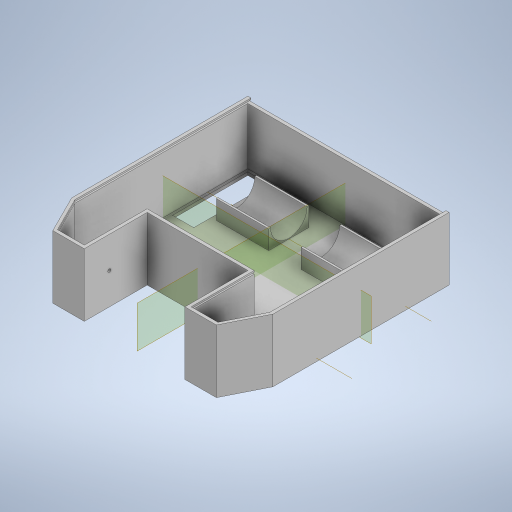
# Autodesk Inventor part: Bot v1 bottom
Saved by Autodesk Inventor 2024 (Build 280153000, 153)
## iProperties
Created: 2023-09-24
Part Number: Bot v1 bottom
Material: PBT Plastic
Document SubType Name: Modeling
Designer: CJ110
Density: 1.31 g/cm^3
Appearance: Smooth - White
Mass: 388.228 g
Surface Area: 1967.58 cm^2
Volume: 296.357 cm^3
Author: CJ110
Autodesk Inventor part; units mm, degrees
ref_plane "YZ Plane" through (0, 0, 0) normal (1, 0, 0) x (0, 1, 0)
sketch "Sketch1" plane through (0, 0, 0) normal (0, 1, 0) x (-1, 0, 0)
  line L0 (0, 0) -> (177.8, 0)
  line L1 (177.8, 0) -> (177.8, 203.2)
  line L2 (177.8, 203.2) -> (0, 203.2)
  line L3 (0, 203.2) -> (0, 0)
  dimension "Body_Length" = 177.8
  dimension "Body_Width" = 203.2
  constraints: 8 end point, 2 parallel, 1 horizontal, 1 perpendicular
  measures "Body_Length" distance of L0.start L0.end
  measures "Body_Width" distance of L2.end L0.start
extrude "Base" add sketch "Sketch1" along normal blind 3.175
sketch "Sketch3" plane through (0, 0, 0) normal (0, 1, 0) x (1, 0, 0)
  line L0 (-177.8, 0) -> (-177.8, -203.2) projected
  line L1 (-177.8, -203.2) -> (0, -203.2) projected
  line L2 (0, -203.2) -> (0, 0) projected
  line L3 (0, 0) -> (-177.8, 0) projected
  line L4 (-174.625, -3.175) -> (-3.175, -3.175)
  line L5 (-3.175, -3.175) -> (-3.175, -200.025)
  line L6 (-3.175, -200.025) -> (-174.625, -200.025)
  line L7 (-174.625, -200.025) -> (-174.625, -155.575)
  line L8 (-152.4, -152.4) -> (-152.4, -50.8)
  line L9 (-174.625, -47.625) -> (-174.625, -3.175)
  line L10 (-177.8, 0) -> (-177.8, -203.2) projected
  line L11 (-174.625, -155.575) -> (-149.225, -155.575)
  line L12 (-149.225, -155.575) -> (-149.225, -47.625)
  line L13 (-149.225, -47.625) -> (-174.625, -47.625)
  line L14 (-152.4, -152.4) -> (-177.8, -152.4)
  line L15 (-152.4, -50.8) -> (-177.8, -50.8)
  dimension "Wall_Thickness" = 3.175
  dimension "Cuttout_Width" = 101.6
  dimension "Cuttout_Depth" = 25.4
  dimension "d30" = 3.175
  dimension "d31" = 3.175
  dimension "d32" = 3.175
  dimension "d33" = 3.175
  constraints: 22 end point, 5 perpendicular, 3 point on line, 2 vertical, 1 collinear, 2 other
  measures "Wall_Thickness" distance between parallel lines of L1 L6
  measures "Cuttout_Width" distance of L8.start L8.end
  measures "Cuttout_Depth" distance between parallel lines of L0 L8
  measures "d30" distance between parallel lines of L0 L7
  measures "d31" distance between parallel lines of L11 L14
  measures "d32" distance between parallel lines of L13 L15
  measures "d33" distance between parallel lines of L8 L12
extrude "Wall" add sketch "Sketch3" along normal blind 63.5 contours L3 L2 L1 L0 L14 L8 L15
sketch "Sketch7" plane through (0, 3.175, 0) normal (0, 1, 0) x (1, 0, 0)
  line L0 (-177.8, -50.8) -> (-177.8, -152.4) projected
  line L1 (-177.8, -152.4) -> (-152.4, -152.4) projected
  line L2 (-152.4, -152.4) -> (-152.4, -50.8) projected
  line L3 (-152.4, -50.8) -> (-177.8, -50.8) projected
  point P0 (0, 0)
extrude "Cuttout" cut sketch "Sketch7" against normal through all
sketch "Sketch2" plane through (0, 3.175, 0) normal (0, 1, 0) x (1, 0, 0)
  line L0 (-172.085, -197.485) -> (-95.885, -197.485)
  line L1 (-95.885, -197.485) -> (-95.885, -186.055)
  line L2 (-95.885, -186.055) -> (-172.085, -186.055)
  line L3 (-172.085, -186.055) -> (-172.085, -197.485)
  line L4 (-81.915, -197.485) -> (-5.715, -197.485)
  line L5 (-5.715, -197.485) -> (-5.715, -175.895)
  line L6 (-5.715, -175.895) -> (-81.915, -175.895)
  line L7 (-81.915, -175.895) -> (-81.915, -197.485)
  line L8 (-177.8, 0) -> (-177.8, -203.2) projected
  line L9 (-177.8, -203.2) -> (0, -203.2) projected
  line L10 (0, -203.2) -> (0, 0) projected
  line L11 (-177.8, -101.6) -> (0, -101.6) construction
  line L12 (-172.085, -5.715) -> (-95.885, -5.715)
  line L13 (-95.885, -5.715) -> (-95.885, -17.145)
  line L14 (-95.885, -17.145) -> (-172.085, -17.145)
  line L15 (-172.085, -17.145) -> (-172.085, -5.715)
  line L16 (-81.915, -5.715) -> (-5.715, -5.715)
  line L17 (-5.715, -5.715) -> (-5.715, -27.305)
  line L18 (-5.715, -27.305) -> (-81.915, -27.305)
  line L19 (-81.915, -27.305) -> (-81.915, -5.715)
  line L20 (-88.9, -203.2) -> (-88.9, 0) construction
  line L21 (0, 0) -> (-177.8, 0) projected
  line L22 (-3.175, -200.025) -> (-174.625, -200.025) projected
  line L23 (-174.625, -200.025) -> (-174.625, -155.575) projected
  line L24 (-3.175, -3.175) -> (-3.175, -200.025) projected
  point P0 (-5.715, -186.69)
  point P1 (-5.715, -16.51)
  dimension "Wheel_Hole_Width" = 11.43
  dimension "Wheel_Hole_Diameter" = 76.2
  dimension "d8" = 76.2
  dimension "Driven_Wheel_Width" = 21.59
  dimension "Wheel_Distance_Side" = 2.54
  dimension "d21" = 6.985
  dimension "Wheel_Distance_Front" = 2.54
  dimension "Wheel_Distance_Back" = 2.54
  constraints: 36 end point, 9 symmetric about line, 5 midpoint, 4 parallel, 2 horizontal, 2 perpendicular, 1 collinear
  measures "Wheel_Hole_Width" distance between parallel lines of L0 L2
  measures "Wheel_Hole_Diameter" distance of L0.start L0.end
  measures "d8" distance of L4.start L4.end
  measures "Driven_Wheel_Width" distance between parallel lines of L4 L6
  measures "Wheel_Distance_Side" distance between parallel lines of L22 L0
  measures "d21" distance between parallel lines of L20 L1
  measures "Wheel_Distance_Front" distance between parallel lines of L23 L3
  measures "Wheel_Distance_Back" distance between parallel lines of L24 L5
extrude "Wheels" cut sketch "Sketch2" against normal up to next contours L3 L2 L1 L0 | L7 L6 L5 L4 | L12 L13 L14 L15 | L16 L17 L18 L19
ref_plane "Work Plane2" through (0, 0, 101.6) normal (0, 0, -1) x (-1, 0, 0)
ref_plane "Work Plane3" through (-88.9, 0, 203.2) normal (1, 0, 0) x (0, 0, -1)
sketch "Sketch11" plane through (0, 63.5, 0) normal (0, 1, 0) x (1, 0, 0)
  line L0 (-174.625, -47.625) -> (-174.625, -3.175) projected
  line L1 (-177.8, 0) -> (-177.8, -203.2) projected
  line L2 (-174.625, -3.175) -> (-177.8, -3.175)
  line L3 (-177.8, -3.175) -> (-177.8, -47.625)
  line L4 (-177.8, -47.625) -> (-174.625, -47.625)
  line L5 (-174.625, -47.625) -> (-174.625, -3.175)
  line L6 (-149.225, -155.575) -> (-174.625, -155.575) projected
  line L7 (-177.8, -152.4) -> (-177.8, -203.2) projected
  line L8 (-174.625, -155.575) -> (-177.8, -155.575)
  line L9 (-177.8, -155.575) -> (-177.8, -200.025)
  line L10 (-177.8, -200.025) -> (-174.625, -200.025)
  line L11 (-174.625, -200.025) -> (-174.625, -155.575)
  line L12 (-149.225, -47.625) -> (-174.625, -47.625) projected
  line L13 (-3.175, -200.025) -> (-174.625, -200.025) projected
  point P0 (0, 0)
  point P1 (-203.2, -50.8)
  constraints: 16 end point, 4 parallel, 2 collinear, 2 horizontal, 2 perpendicular, 1 point on line, 2 other
extrude "Extrusion11" cut sketch "Sketch11" against normal up to surface (60.325 mm away)
sketch "Sketch12" plane through (0, 0, 0) normal (0, -1, 0) x (1, 0, 0)
  line L0 (-172.085, 17.145) -> (-95.885, 17.145) projected
  line L1 (-95.885, 17.145) -> (-95.885, 5.715) projected
  line L2 (-95.885, 5.715) -> (-172.085, 5.715) projected
  line L3 (-172.085, 5.715) -> (-172.085, 17.145) projected
  line L4 (-5.715, 175.895) -> (-81.915, 175.895) projected
  line L5 (-81.915, 175.895) -> (-81.915, 197.485) projected
  line L6 (-81.915, 197.485) -> (-5.715, 197.485) projected
  line L7 (-5.715, 197.485) -> (-5.715, 175.895) projected
  line L8 (-5.715, 27.305) -> (-5.715, 5.715) projected
  line L9 (-5.715, 5.715) -> (-81.915, 5.715) projected
  line L10 (-81.915, 5.715) -> (-81.915, 27.305) projected
  line L11 (-81.915, 27.305) -> (-5.715, 27.305) projected
  line L12 (-95.885, 186.055) -> (-172.085, 186.055) projected
  line L13 (-172.085, 186.055) -> (-172.085, 197.485) projected
  line L14 (-172.085, 197.485) -> (-95.885, 197.485) projected
  line L15 (-95.885, 197.485) -> (-95.885, 186.055) projected
  line L16 (-152.4, 50.8) -> (-177.8, 50.8) projected
  line L17 (-177.8, 0) -> (-177.8, 50.8) projected
  line L18 (0, 0) -> (-177.8, 0) projected
  line L19 (0, 203.2) -> (0, 0) projected
  line L20 (-177.8, 203.2) -> (0, 203.2) projected
  line L21 (-177.8, 152.4) -> (-177.8, 203.2) projected
  line L22 (-177.8, 152.4) -> (-152.4, 152.4) projected
  line L23 (-152.4, 152.4) -> (-152.4, 50.8) projected
  line L24 (-3.175, 200.025) -> (-177.8, 200.025) projected
  line L25 (-177.8, 200.025) -> (-177.8, 203.2) projected
  line L26 (-177.8, 203.2) -> (0, 203.2) projected
  line L27 (0, 203.2) -> (0, 0) projected
  line L28 (0, 0) -> (-177.8, 0) projected
  line L29 (-177.8, 0) -> (-177.8, 3.175) projected
  line L30 (-177.8, 3.175) -> (-3.175, 3.175) projected
  line L31 (-3.175, 3.175) -> (-3.175, 200.025) projected
  line L32 (-177.8, 155.575) -> (-149.225, 155.575) projected
  line L33 (-149.225, 155.575) -> (-149.225, 47.625) projected
  line L34 (-149.225, 47.625) -> (-177.8, 47.625) projected
  line L35 (-177.8, 47.625) -> (-177.8, 50.8) projected
  line L36 (-177.8, 50.8) -> (-152.4, 50.8) projected
  line L37 (-152.4, 50.8) -> (-152.4, 152.4) projected
  line L38 (-152.4, 152.4) -> (-177.8, 152.4) projected
  line L39 (-177.8, 152.4) -> (-177.8, 155.575) projected
  line L40 (-177.8, 0) -> (-215.9, 19.05)
  line L41 (-215.9, 19.05) -> (-215.9, 50.8)
  line L42 (-215.9, 50.8) -> (-177.8, 50.8)
  line L43 (-177.8, 3.175) -> (-212.725, 20.6375)
  line L44 (-212.725, 20.6375) -> (-212.725, 47.625)
  line L45 (-212.725, 47.625) -> (-177.8, 47.625)
  line L46 (-152.4, 50.8) -> (-152.4, 152.4) projected
  line L47 (-152.4, 101.6) -> (0, 101.6) construction
  line L48 (-177.8, 203.2) -> (-215.9, 184.15)
  line L49 (-215.9, 184.15) -> (-215.9, 152.4)
  line L50 (-215.9, 152.4) -> (-177.8, 152.4)
  line L51 (-177.8, 200.025) -> (-212.725, 182.5625)
  line L52 (-212.725, 182.5625) -> (-212.725, 155.575)
  line L53 (-212.725, 155.575) -> (-177.8, 155.575)
  line L54 (-95.885, 17.145) -> (-172.085, 17.145) projected
  line L55 (-172.085, 17.145) -> (-172.085, 5.715) projected
  line L56 (-172.085, 5.715) -> (-95.885, 5.715) projected
  line L57 (-95.885, 5.715) -> (-95.885, 17.145) projected
  line L58 (-81.915, 175.895) -> (-5.715, 175.895) projected
  line L59 (-5.715, 175.895) -> (-5.715, 197.485) projected
  line L60 (-5.715, 197.485) -> (-81.915, 197.485) projected
  line L61 (-81.915, 197.485) -> (-81.915, 175.895) projected
  line L62 (-5.715, 5.715) -> (-5.715, 27.305) projected
  line L63 (-5.715, 27.305) -> (-81.915, 27.305) projected
  line L64 (-81.915, 27.305) -> (-81.915, 5.715) projected
  line L65 (-81.915, 5.715) -> (-5.715, 5.715) projected
  line L66 (-172.085, 186.055) -> (-95.885, 186.055) projected
  line L67 (-95.885, 186.055) -> (-95.885, 197.485) projected
  line L68 (-95.885, 197.485) -> (-172.085, 197.485) projected
  line L69 (-172.085, 197.485) -> (-172.085, 186.055) projected
  line L70 (-177.8, 47.625) -> (-149.225, 47.625) projected
  line L71 (-149.225, 47.625) -> (-149.225, 155.575) projected
  line L72 (-149.225, 155.575) -> (-177.8, 155.575) projected
  line L73 (-177.8, 200.025) -> (-177.8, 155.575) projected
  line L74 (-177.8, 200.025) -> (-3.175, 200.025) projected
  line L75 (-3.175, 200.025) -> (-3.175, 3.175) projected
  line L76 (-177.8, 3.175) -> (-3.175, 3.175) projected
  line L77 (-177.8, 47.625) -> (-177.8, 3.175) projected
  point P0 (-203.2, 155.575)
  point P1 (-203.2, 200.025)
  point P2 (-203.2, 152.4)
  point P3 (-203.2, 203.2)
  point P4 (-203.2, 3.175)
  point P5 (-203.2, 47.625)
  point P6 (-203.2, 200.025)
  point P7 (-203.2, 3.175)
  point P8 (-203.2, 155.575)
  point P9 (-203.2, 47.625)
  point P10 (-203.2, 50.8)
  point P11 (-203.2, 0)
  dimension "d52" = 3.175
  dimension "d53" = 38.1
  dimension "d54" = 31.75
  constraints: 26 end point, 6 symmetric about line, 2 horizontal, 2 midpoint, 2 parallel, 1 vertical
  measures "d52" distance between parallel lines of L41 L44
  measures "d53" distance between parallel lines of L17 L41
  measures "d54" distance of L40.end L41.end
extrude "Extrusion12" add sketch "Sketch12" against normal up to surface (3.175 mm away) contours L17 L45 L44 L43 L40 L41 L42 | L17 L43 L44 L45 | L50 L49 L48 L21 L51 L52 L53 | L53 L52 L51 L21
extrude "Extrusion13" add sketch "Sketch12" against normal up to surface (63.5 mm away) contours L17 L45 L44 L43 L40 L41 L42 | L50 L49 L48 L21 L51 L52 L53
ref_plane "Work Plane4" through (0, 31.75, 0) normal (0, -1, 0) x (1, 0, 0)
sketch "Sketch13" plane through (-152.4, 0, 50.8) normal (0, 0, 1) x (1, 0, 0)
  line L0 (0, 0) -> (-63.5, 0) projected
  line L1 (0, 63.5) -> (0, 0) projected
  line L2 (0, 63.5) -> (-63.5, 63.5)
  line L3 (-63.5, 0) -> (-63.5, 63.5) projected
  line L4 (-63.5, 63.5) -> (0, 63.5)
  circle A0 centre (-38.1, 31.75) radius 1.55
  line L5 (195.58, 31.75) -> (-106.68, 31.75) projected
  point P0 (152.4, 0)
  point P1 (-33.3, 76.2)
  point P2 (-30.2, 76.2)
  dimension "d59" = 3.1
  dimension "d74" = 25.4
  constraints: 4 end point, 1 centre point, 1 point on line
  measures "d59" diameter of A0
  measures "d74" distance from line of L3 A0.centre
extrude "Extrusion14" cut sketch "Sketch13" against normal up to surface (3.175 mm away) contours L5 A0 | A0 L5
sketch "Sketch15" plane through (0, 0, 203.2) normal (1, 0, 0) x (0, 0, -1)
  line L0 (0, 63.5) -> (19.05, 63.5) projected
  line L1 (3.175, 63.5) -> (200.025, 63.5)
  line L2 (200.025, 63.5) -> (200.025, 60.325)
  line L3 (200.025, 60.325) -> (3.175, 60.325)
  line L4 (3.175, 60.325) -> (3.175, 63.5)
  line L5 (243.84, 31.75) -> (-40.64, 31.75) projected
  line L6 (3.175, 3.175) -> (200.025, 3.175) projected
  line L7 (3.175, 3.175) -> (3.175, 63.5) projected
  line L8 (200.025, 63.5) -> (3.175, 63.5) projected
  line L9 (200.025, 3.175) -> (200.025, 63.5) projected
  point P0 (203.2, 0)
  point P1 (19.05, 63.5)
  dimension "d75" = 3.175
  constraints: 8 end point, 2 collinear, 2 parallel, 1 horizontal, 1 perpendicular, 1 point on line
  measures "d75" distance between parallel lines of L3 L1
extrude "Extrusion16" cut sketch "Sketch15" against normal up to surface (3.175 mm away) contours L0 L1 L2 L3 L4
ref_plane "Work Plane5" through (0, 60.325, 200.025) normal (0, 1, 0) x (1, 0, 0)
sketch "Sketch17" plane through (0, 60.325, 200.025) normal (0, 1, 0) x (1, 0, 0)
  line L0 (-177.8, 196.85) -> (-3.175, 196.85) projected
  line L1 (0, 196.85) -> (-3.175, 196.85) projected
  line L2 (-177.8, 196.85) -> (0, 196.85) projected
  line L3 (-177.8, 0) -> (-3.175, 0) projected
  line L4 (0, 0) -> (-177.8, 0) projected
  line L5 (0, 0) -> (-3.175, 0) projected
  line L6 (-212.725, 17.4625) -> (-177.8, 0) projected
  line L7 (-212.725, 17.4625) -> (-177.8, 0) projected
  line L8 (-212.725, 44.45) -> (-212.725, 17.4625) projected
  line L9 (-212.725, 44.45) -> (-212.725, 17.4625) projected
  line L10 (-177.8, 196.85) -> (-212.725, 179.3875) projected
  line L11 (-149.225, 44.45) -> (-212.725, 44.45) projected
  line L12 (-212.725, 44.45) -> (-149.225, 44.45) projected
  line L13 (-149.225, 152.4) -> (-149.225, 44.45) projected
  line L14 (-149.225, 44.45) -> (-149.225, 152.4) projected
  line L15 (-212.725, 179.3875) -> (-212.725, 152.4) projected
  line L16 (-212.725, 179.3875) -> (-212.725, 152.4) projected
  line L17 (-192.05, 152.4) -> (-188.95, 152.4) projected
  line L18 (-212.725, 152.4) -> (-149.225, 152.4) projected
  line L19 (-212.725, 152.4) -> (-149.225, 152.4) projected
  line L20 (0, -3.175) -> (0, 200.025) projected
  line L21 (0, -1.5875) -> (-177.8, -1.5875)
  line L22 (-177.8, -1.5875) -> (-214.3125, 16.6688)
  line L23 (-177.8, -3.175) -> (-215.9, 15.875) projected
  line L24 (-214.3125, 16.6688) -> (-214.3125, 46.0375)
  line L25 (-214.3125, 46.0375) -> (-150.8125, 46.0375)
  line L26 (-150.8125, 46.0375) -> (-150.8125, 150.8125)
  line L27 (-150.8125, 150.8125) -> (-214.3125, 150.8125)
  line L28 (-214.3125, 150.8125) -> (-214.3125, 180.1813)
  line L29 (-214.3125, 180.1813) -> (-177.8, 198.4375)
  line L30 (-177.8, 198.4375) -> (0, 198.4375)
  line L31 (-212.725, 179.3875) -> (-215.9, 180.975) construction
  line L32 (-177.8, 196.85) -> (-177.8, 200.025) construction
  line L33 (-152.4, 149.225) -> (-215.9, 149.225) projected
  line L34 (-212.725, 152.4) -> (-215.9, 149.225) construction
  line L35 (-152.4, 149.225) -> (-149.225, 152.4) construction
  line L36 (-152.4, 47.625) -> (-152.4, 149.225) construction
  line L37 (-152.4, 47.625) -> (-149.225, 44.45) construction
  line L38 (-215.9, 47.625) -> (-152.4, 47.625) construction
  line L39 (-212.725, 44.45) -> (-215.9, 47.625) construction
  line L40 (-212.725, 17.4625) -> (-215.9, 15.875) construction
  line L41 (-177.8, -3.175) -> (-177.8, 0) construction
  line L42 (-177.8, -3.175) -> (0, -3.175) construction
  line L43 (-177.8, 196.85) -> (-212.725, 179.3875) projected
  point P0 (-3.175, 0)
  point P1 (-3.175, 196.85)
  point P2 (0, 198.4375)
  dimension "d87" = 1.5875
  dimension "d88" = 1.5875
  constraints: 34 end point, 8 midpoint, 4 parallel, 4 perpendicular, 1 horizontal, 1 point on line, 1 vertical
  measures "d87" distance of L1.start L30.end
  measures "d88" distance of L0.start L29.end
extrude "Extrusion17" cut sketch "Sketch17" along normal blind 1.5875
sketch "Sketch20" plane through (0, 3.175, 0) normal (0, 1, 0) x (1, 0, 0)
  line L0 (-64.135, -32.385) -> (-23.495, -32.385)
  line L1 (-23.495, -32.385) -> (-23.495, -85.217)
  line L2 (-23.495, -85.217) -> (-64.135, -85.217)
  line L3 (-64.135, -85.217) -> (-64.135, -32.385)
  line L4 (-5.715, -27.305) -> (-81.915, -27.305) projected
  line L5 (-43.815, -243.84) -> (-43.815, 40.64) projected
  line L6 (-212.725, -47.625) -> (-149.225, -47.625) projected
  line L7 (-149.225, -47.625) -> (-149.225, -155.575) projected
  line L8 (-149.225, -155.575) -> (-212.725, -155.575) projected
  line L9 (-212.725, -155.575) -> (-212.725, -182.5625) projected
  line L10 (-212.725, -182.5625) -> (-177.8, -200.025) projected
  line L11 (-177.8, -200.025) -> (-3.175, -200.025) projected
  line L12 (-3.175, -200.025) -> (-3.175, -3.175) projected
  line L13 (-177.8, -3.175) -> (-3.175, -3.175) projected
  line L14 (-177.8, -3.175) -> (-212.725, -20.6375) projected
  line L15 (-212.725, -20.6375) -> (-212.725, -47.625) projected
  line L16 (-95.885, -17.145) -> (-172.085, -17.145) projected
  line L17 (-172.085, -17.145) -> (-172.085, -5.715) projected
  line L18 (-172.085, -5.715) -> (-95.885, -5.715) projected
  line L19 (-95.885, -5.715) -> (-95.885, -17.145) projected
  line L20 (-81.915, -175.895) -> (-5.715, -175.895) projected
  line L21 (-5.715, -175.895) -> (-5.715, -197.485) projected
  line L22 (-5.715, -197.485) -> (-81.915, -197.485) projected
  line L23 (-81.915, -197.485) -> (-81.915, -175.895) projected
  line L24 (-5.715, -5.715) -> (-5.715, -27.305) projected
  line L25 (-5.715, -27.305) -> (-81.915, -27.305) projected
  line L26 (-81.915, -27.305) -> (-81.915, -5.715) projected
  line L27 (-81.915, -5.715) -> (-5.715, -5.715) projected
  line L28 (-172.085, -186.055) -> (-95.885, -186.055) projected
  line L29 (-95.885, -186.055) -> (-95.885, -197.485) projected
  line L30 (-95.885, -197.485) -> (-172.085, -197.485) projected
  line L31 (-172.085, -197.485) -> (-172.085, -186.055) projected
  line L32 (-149.225, -101.6) -> (-3.175, -101.6) construction
  line L33 (-64.135, -170.815) -> (-23.495, -170.815)
  line L34 (-23.495, -170.815) -> (-23.495, -117.983)
  line L35 (-23.495, -117.983) -> (-64.135, -117.983)
  line L36 (-64.135, -117.983) -> (-64.135, -170.815)
  point P0 (0, 0)
  dimension "d92" = 5.08
  dimension "d93" = 40.64
  dimension "d95" = 52.832
  dimension "d101" = 20.32
  constraints: 18 end point, 4 symmetric about line, 2 midpoint, 2 parallel, 1 horizontal, 1 perpendicular
  measures "d92" distance between parallel lines of L4 L0
  measures "d93" distance between parallel lines of L3 L1
  measures "d95" distance between parallel lines of L0 L2
  measures "d101" distance between parallel lines of L3 L5
extrude "Extrusion18" add sketch "Sketch20" along normal blind 19.05 contours L0 L5 L2 L3 | L0 L1 L2 L5 | L35 L34 L33 L5 | L5 L33 L36 L35
sketch "Sketch22" plane through (0, 0, 101.6) normal (0, 0, -1) x (-1, 0, 0)
  line L0 (64.135, 22.225) -> (23.495, 22.225) projected
  arc A0 (25.3365, 22.225) -> (62.2935, 22.225) centre (43.815, 22.225) ccw
  line L1 (23.495, 3.175) -> (64.135, 3.175) projected
  line L2 (23.495, 3.175) -> (23.495, 22.225) projected
  line L3 (64.135, 22.225) -> (23.495, 22.225) projected
  line L4 (64.135, 3.175) -> (64.135, 22.225) projected
  point P0 (0, 0)
  dimension "d98" = 36.957
  constraints: 2 point on circle, 2 point on line, 1 centre point, 1 midpoint
  measures "d98" diameter of A0
extrude "Extrusion19" cut sketch "Sketch22" along normal mid plane 139.7 contours A0 L0
equation "\"Bottom_Thickness\" = Wall_Thickness"
equation "\"d30\" = Wall_Thickness"
equation "\"d31\" = Wall_Thickness"
equation "\"d32\" = Wall_Thickness"
equation "\"d33\" = Wall_Thickness"
equation "\"d8\" = Wheel_Hole_Diameter"
equation "\"Wheel_Distance_Front\" = Wheel_Distance_Back"
equation "\"d52\" = Wall_Thickness"
equation "\"d75\" = Wall_Thickness"
equation "\"d87\" = 0.5 * Wall_Thickness"
equation "\"d89\" = 0.5 * Wall_Thickness"
equation "\"d101\" = 0.5 * d93"
equation "\"d72\" = -0.5 * Wall_Height"
equation "\"Wall_Height\" = 63.5"
body "Solid1"
